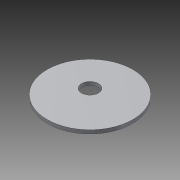
# Autodesk Inventor part: cooling_element
Saved by Autodesk Inventor 2014 (Build 180170000, 170)
## iProperties
Created: 2014-03-25
Part Number: cooling_element
Material: Aluminum 6061
Document SubType Name: Modeling
Designer: buben
Density: 2.71 g/cm^3
Appearance: Aluminum - Flat
Mass: 1.28772 g
Surface Area: 10.4491 cm^2
Volume: 0.475174 cm^3
Author: buben
Autodesk Inventor part; units mm, degrees
ref_plane "YZ Plane" through (0, 0, 0) normal (1, 0, 0) x (0, 1, 0)
ref_plane "XZ Plane" through (0, 0, 0) normal (0, 1, 0) x (-1, 0, 0)
ref_plane "XY Plane" through (0, 0, 0) normal (0, 0, 1) x (1, 0, 0)
sketch "Sketch1" plane through (0, 0, 0) normal (0, 0, 1) x (1, 0, 0)
  circle A0 centre (0, 0) radius 12.55
  circle A1 centre (0, 0) radius 2.5
  dimension "d0" = 25.1
  dimension "d1" = 5
  constraints: 2 centre point, 2 coincident
  measures "d0" diameter of A0
  measures "d1" diameter of A1
extrude "Extrusion1" add sketch "Sketch1" along normal blind 1
body "Solid1"
